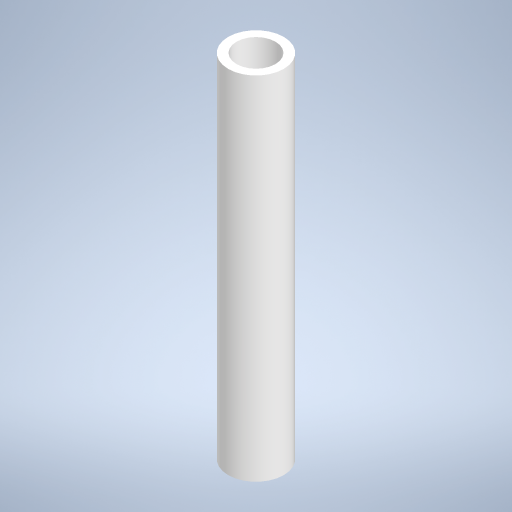
# Autodesk Inventor part: Distanz
Saved by Autodesk Inventor 2024.4 (Build 284460000, 460)
## iProperties
Created: 2026-01-14
Part Number: Distanz
Material: PVC, hart
Description: Distanz
Document SubType Name: Modeling
Designer: Philf
Mass: 88.358 g
Surface Area: 311.63 cm^2
Volume: 68.4946 cm^3
Density: 1.29 g/cm^3
Appearance: Glatt - Weiß
Masse[kg]: 0,068 kg
Author: Philf
Autodesk Inventor part; units mm, degrees
ref_plane "YZ Plane" through (0, 0, 0) normal (1, 0, 0) x (0, 1, 0)
ref_plane "XZ Plane" through (0, 0, 0) normal (0, 1, 0) x (-1, 0, 0)
ref_plane "XY Plane" through (0, 0, 0) normal (0, 0, 1) x (1, 0, 0)
sketch "Skizze1" plane through (0, 0, 0) normal (0, 0, 1) x (1, 0, 0)
  circle A0 centre (0, 0) radius 15
  circle A1 centre (0, 0) radius 10.5
  dimension "außendurchmesser" = 30
  dimension "innendurchmesser" = 21
  constraints: 2 centre point, 2 coincident
  measures "außendurchmesser" diameter of A0
  measures "innendurchmesser" diameter of A1
extrude "Extrusion1" add sketch "Skizze1" along normal blind 190
